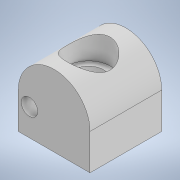
# Autodesk Inventor part: pist
Saved by Autodesk Inventor 2022 (Build 260153000, 153)
## iProperties
Created: 2022-12-19
Part Number: pist
Material: Generic
Document SubType Name: Modeling
Designer: matys
Density: 1 g/cm^3
Appearance: Default
Author: matys
Autodesk Inventor part; units mm, degrees
ref_plane "YZ Plane" through (0, 0, 0) normal (1, 0, 0) x (0, 1, 0)
ref_plane "XZ Plane" through (0, 0, 0) normal (0, 1, 0) x (-1, 0, 0)
ref_plane "XY Plane" through (0, 0, 0) normal (0, 0, 1) x (1, 0, 0)
sketch "Sketch1" plane through (0, 0, 0) normal (0, 1, 0) x (-1, 0, 0)
  line L0 (0, 0) -> (0, -4.2)
  circle A0 centre (0, -2.1) radius 2.1
  line L1 (0, -2.1) -> (0, -6.9)
  line L2 (0, -6.9) -> (0, 2.7)
  line L3 (0, 2.7) -> (5, 2.7)
  line L4 (5, 2.7) -> (5, -7.3)
  line L5 (5, -7.3) -> (-5, -7.3)
  line L6 (-5, -7.3) -> (-5, 2.7)
  line L7 (-5, 2.7) -> (0, 2.7)
  dimension "d0" = 4.2
  dimension "d1" = 4.8
  dimension "d2" = 9.6
  dimension "d3" = 5
  dimension "d4" = 10
  constraints: 16 end point, 4 perpendicular, 2 point on line, 2 vertical, 1 horizontal, 1 midpoint, 1 vertical alignment, 2 other
  measures "d0" distance of L0.start L0.end
  measures "d1" distance of L1.start L1.end
  measures "d2" distance of L1.end L2.end
  measures "d3" distance of L2.end L3.end
  measures "d4" distance of L4.end L5.end
extrude "Extrusion1" add sketch "Sketch1" along normal blind 10
sketch "Sketch2" plane through (0, 10, 0) normal (0, 1, 0) x (1, 0, 0)
  circle A0 centre (0, 2.1) radius 2.1 projected
  circle A1 centre (0, 2.1) radius 3
  point P0 (0, 0)
  dimension "d7" = 6
  constraints: 1 centre point, 1 coincident, 1 vertical alignment
  measures "d7" diameter of A1
extrude "Extrusion2" cut sketch "Sketch2" against normal blind 3.5 contours A0 | A1
fillet "Fillet1" radius 5 2 edges at (5, 10, -2.3) (-5, 10, -2.3)
sketch "Sketch3" plane through (-5, 0, 2.7) normal (0, 0, 1) x (1, 0, 0)
  arc A0 (10, 5) -> (0, 5) centre (5, 5) ccw projected
  line L0 (5, 5) -> (5, 10)
  line L1 (5, 5) -> (5, 0)
  line L2 (5, 0) -> (5, 5)
  line L3 (0, 0) -> (0, 5) projected
  line L4 (5, 5) -> (0, 5)
  line L5 (0, 5) -> (2.5, 5)
  line L6 (2.5, 5) -> (2.5, 0)
  line L7 (2.5, 0) -> (2.5, 2.5)
  line L8 (1.25, 5) -> (1.25, 0)
  line L9 (0, 0) -> (10, 0) projected
  line L10 (2.5, 2.5) -> (1.25, 2.5)
  line L11 (1.875, 5) -> (1.875, 2.5)
  circle A1 centre (1.875, 2.5) radius 1.15
  line L12 (1.25, 5) -> (1.875, 5)
  line L13 (1.5625, 5) -> (1.5625, 2.5)
  line L14 (1.5625, 2.5) -> (1.5625, 3.75)
  circle A2 centre (1.5625, 3.75) radius 1.15
  line L15 (1.5625, 3.75) -> (0.4125, 3.75)
  line L16 (0.4125, 3.75) -> (0, 3.75)
  dimension "d14" = 2.3
  constraints: 30 end point, 7 midpoint, 5 point on line, 4 vertical, 3 coincident, 2 collinear, 2 horizontal, 1 centre point, 1 horizontal alignment, 1 perpendicular, 1 point on circle, 2 other
extrude "Extrusion3" cut sketch "Sketch3" against normal through all contours L15 L8 A1 A2 | A2 L8 L15 | A2 L13 L15 L8 | A2 A1 L6 | L6 A1 L11 A2 | A1 L8 A2 | L15 L13 A1 L8 | A2 L11 A1 L13 | A1 A2 L6 | L6 A2 L11 A1 | A1 L13 A2 L8 | L11 A2 L13 A1 picked at (2.5388, 4.0306) picked at (1.186, 3.1393) picked at (2.5186, 3.2399)
body "Solid1"
